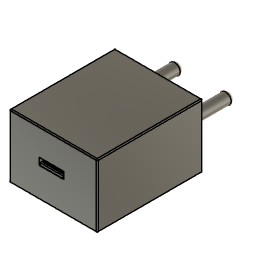
Day 2 Charger v1 (Autodesk Fusion 360 design; units mm, degrees)
Autodesk Fusion 360 part; units mm, degrees
sketch "Sketch1" plane through (0, 0, 0) normal (0, 1, 0) x (1, 0, 0)
  line L0 (0, 0) -> (50, 0)
  line L1 (50, 0) -> (50, -50)
  line L2 (50, -50) -> (0, -50)
  line L3 (0, -50) -> (0, 0)
  constraint horizontal L0
  constraint vertical L1
  constraint horizontal L2
  constraint vertical L3
  constraint coincident L0.start L3.end
extrude "Extrude1" add sketch "Sketch1" along normal blind 60
move_face "MoveFace1" by (-1.5603, -0.957, -13.7498) 1 faces at (33.3333, 40, 50)
sketch "Sketch2" plane through (0, 60, 0) normal (0, 1, 0) x (-1, 0, 0)
  line L0 (0, 36.2502) -> (-50, 36.2502)
  line L1 (-50, 36.2502) -> (-50, 0)
  line L2 (-50, 0) -> (0, 0)
  line L3 (0, 0) -> (0, 36.2502)
  circle A0 centre (-40, 20) radius 3.1623
  point P0 (-22, 20)
extrude "Extrude2" add sketch "Sketch2" along normal blind 25 contours A0
fillet "Fillet1" radius 2 1 edges at (42.9483, 85, 18.8565)
pattern_linear "R-Pattern1" count 2 spacing 29 along (-1, 0, 0) of "Extrude2"
fillet "Fillet2" radius 2 1 faces at (9.1218, 85, 19.0955)
sketch "Sketch3" plane through (0, 0, 0) normal (0, -1, 0) x (1, 0, 0)
  line L0 (50, 36.2502) -> (0, 36.2502)
  line L1 (0, 36.2502) -> (0, 0)
  line L2 (0, 0) -> (50, 0)
  line L3 (50, 0) -> (50, 36.2502)
  line L4 (17, 21) -> (31, 21)
  line L5 (31, 21) -> (31, 17)
  line L6 (31, 17) -> (17, 17)
  line L7 (17, 17) -> (17, 21)
  constraint horizontal L4
  constraint vertical L5
  constraint horizontal L6
  constraint vertical L7
extrude "Extrude3" cut sketch "Sketch3" against normal blind 14 contours L4 L5 L6 L7
sketch "Sketch4" plane through (0, 14, 0) normal (0, -1, 0) x (1, 0, 0)
  line L0 (17, 17) -> (31, 17)
  line L1 (31, 17) -> (31, 21)
  line L2 (31, 21) -> (17, 21)
  line L3 (17, 21) -> (17, 17)
  line L4 (17.5, 18.5) -> (30.5682, 18.5)
  line L5 (30.5682, 18.5) -> (30.5682, 17.1968)
  line L6 (30.5682, 17.1968) -> (17.5, 17.1968)
  line L7 (17.5, 17.1968) -> (17.5, 18.5)
  constraint horizontal L4
  constraint vertical L5
  constraint horizontal L6
  constraint vertical L7
extrude "Extrude4" add sketch "Sketch4" along normal blind 14 contours L4 L5 L6 L7
sketch "Sketch5" plane through (0, 0, 18.5) normal (0, 0, 1) x (-1, 0, 0)
  line L0 (-30.5682, -14) -> (-17.5, -14)
  line L1 (-17.5, -14) -> (-17.5, 0)
  line L2 (-17.5, 0) -> (-30.5682, 0)
  line L3 (-30.5682, 0) -> (-30.5682, -14)
  line L4 (-18.1742, -14) -> (-18.5, -14)
  line L5 (-18.5, -14) -> (-18.5, -1)
  line L6 (-18.5, -1) -> (-18.1742, -1)
  line L7 (-18.1742, -1) -> (-18.1742, -14)
  constraint horizontal L4
  constraint vertical L5
  constraint horizontal L6
  constraint vertical L7
  constraint coincident L0 L4.start
extrude "Extrude5" cut sketch "Sketch5" against normal blind 0.1 contours L0 L4 L5 L6 L7
pattern_linear "R-Pattern2" count 25 spacing 0.4792 along (1, 0, 0) of "Extrude5"
fillet "Fillet3" radius 0.6 5 edges at (50, 0, 18.1251) (50, 30, 36.2502) (25, 0, 36.2502) (50, 30, 0) (25, 0, 0)
fillet "Fillet4" radius 0.6 11 edges at (24.7, 60, 36.2502) (49.8243, 60, 36.0745) (50, 60, 18.1251) (49.8243, 60, 0.1757) (24.7, 60, 0) (0, 60, 18.1251) (0, 30.3, 36.2502) (0, 0.1757, 36.0745) (0, 0, 18.1251) (0, 0.1757, 0.1757) (0, 30.3, 0)
sketch "Sketch6" plane through (0, 0, 0) normal (-1, 0, 0) x (0, -1, 0)
  line L0 (-0.6, 0.6) -> (-0.6, 35.6502)
  line L1 (-0.6, 35.6502) -> (-59.4, 35.6502)
  line L2 (-59.4, 35.6502) -> (-59.4, 0.6)
  line L3 (-59.4, 0.6) -> (-0.6, 0.6)
  line L4 (-41, 18) -> (-14, 18) construction
  line L5 (-14, 18) -> (-14, 27) construction
  line L6 (-14, 27) -> (-41, 27) construction
  line L7 (-41, 27) -> (-41, 18) construction
  dimension "d27" = 2
  text T0 "Unknow Charger" font "Arial" height 2 align left top in box 27 x 9 at (-41, 18) x (1, 0) y (0, 1) spacing 1
extrude "Extrude6" cut sketch "Sketch6" against normal blind 0.6 text T0
